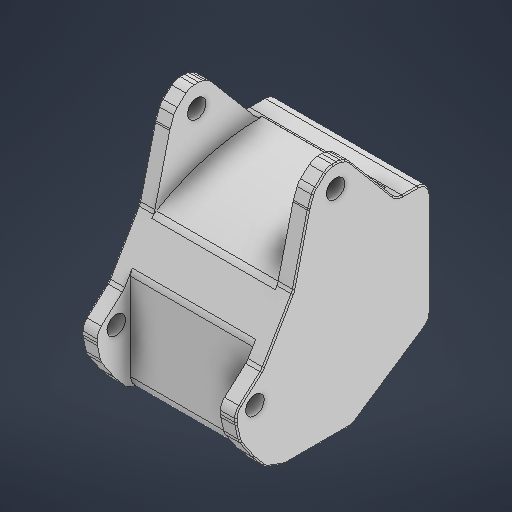
# Autodesk Inventor part: bas
Saved by Autodesk Inventor 2026 (Build 300175000, 175)
## iProperties
Created: 2025-04-29
Part Number: bas
Material: Generic
Document SubType Name: Modeling
Designer: elias
Density: 1 g/cm^3
Appearance: Default
Author: elias
Autodesk Inventor part; units mm, degrees
ref_plane "YZ Plane" through (0, 0, 0) normal (1, 0, 0) x (0, 1, 0)
ref_plane "XZ Plane" through (0, 0, 0) normal (0, 1, 0) x (-1, 0, 0)
ref_plane "XY Plane" through (0, 0, 0) normal (0, 0, 1) x (1, 0, 0)
sketch "Sketch1" plane through (0, 0, 0) normal (1, 0, 0) x (0, 1, 0)
  line L0 (3056.2025, 0) -> (3056.2025, -6694.5386) construction
  line L1 (3056.2025, -6694.5386) -> (0, -6694.5386) construction
  line L2 (0, -6694.5386) -> (0, 0) construction
  line L3 (0, 0) -> (3056.2025, 0) construction
  point P0 (0, 0)
  constraints: 2 end point, 2 other
sketch "Sketch3" plane through (0, 0, 0) normal (1, 0, 0) x (0, 1, 0)
  line L0 (685.9944, -4625.4625) -> (724.6137, -4668.6643)
  line L1 (724.6137, -4668.6643) -> (809.1123, -4718.3258)
  line L2 (809.1123, -4718.3258) -> (912.0878, -4743.403)
  line L3 (912.0878, -4743.403) -> (934.1067, -4751.4736)
  line L4 (934.1067, -4751.4736) -> (945.5061, -4764.2256)
  line L5 (945.5061, -4764.2256) -> (955.4629, -4775.3639)
  line L6 (955.4629, -4775.3639) -> (955.4629, -4793.4979)
  line L7 (955.4629, -4793.4979) -> (950.4845, -4807.0804)
  line L8 (950.4845, -4807.0804) -> (855.8729, -4886.5328)
  line L9 (855.8729, -4886.5328) -> (855.8729, -4940.715)
  line L10 (855.8729, -4940.715) -> (817.0202, -4940.715)
  line L11 (817.0202, -4940.715) -> (659.1622, -4940.715)
  line L12 (659.1622, -4940.715) -> (574.4497, -4814.0948)
  line L13 (574.4497, -4814.0948) -> (574.4497, -4703.7938)
  line L14 (574.4497, -4703.7938) -> (585.6108, -4673.3431)
  line L15 (585.6108, -4673.3431) -> (609.1892, -4653.5426)
  line L16 (609.1892, -4653.5426) -> (641.8589, -4631.6856)
  line L17 (641.8589, -4631.6856) -> (669.5109, -4625.4625)
  line L18 (669.5109, -4625.4625) -> (685.9944, -4625.4625)
  circle A0 centre (681.295, -4656.3748) radius 15
  circle A1 centre (920.0279, -4787.0013) radius 15
  point P0 (0, 0)
  dimension "d14" = 30
  dimension "d15" = 30
  constraints: 38 end point, 5 perpendicular, 4 parallel, 2 centre point, 2 point on line, 1 vertical
  measures "d14" diameter of A0
  measures "d15" diameter of A1
extrude "Extrusion1" add sketch "Sketch3" along normal mid plane 250
fillet "Fillet1" radius 20 17 edges at (0, 669.5109, -4625.4625) (0, 685.9944, -4625.4625) (0, 724.6137, -4668.6643) (0, 809.1123, -4718.3258) (0, 912.0878, -4743.403) (0, 934.1067, -4751.4736) (0, 950.4845, -4807.0804) (0, 955.4629, -4793.4979) (0, 955.4629, -4775.3639) (0, 855.8729, -4886.5328) (0, 855.8729, -4940.715) (0, 659.1622, -4940.715) (0, 574.4497, -4814.0948) (0, 641.8589, -4631.6856) (0, 609.1892, -4653.5426) (0, 585.6108, -4673.3431) (0, 574.4497, -4703.7938)
fillet "Fillet2" radius 2 68 edges at (125, 724.7675, -4668.4766) (125, 707.2443, -4649.2338) (125, 685.2143, -4627.2062) (125, 674.3902, -4625.4625) (125, 669.5245, -4625.5849) (125, 656.4177, -4628.4091) (125, 641.9946, -4632.0016) (125, 624.4291, -4643.3467) (125, 609.207, -4653.5663) (125, 599.0237, -4662.0793) (125, 586.1824, -4673.7441) (125, 579.7239, -4689.4044) (125, 574.7575, -4703.8485) (125, 574.4497, -4757.6826) (125, 575.3126, -4813.8328) (125, 615.5244, -4875.4894) (125, 660.4221, -4938.3562) (125, 752.8589, -4940.715) (125, 850.015, -4934.8572) (125, 855.8729, -4908.2846) (125, 857.745, -4887.4053) (125, 904.7067, -4845.5234) (125, 949.913, -4806.6794) (125, 953.2801, -4799.4532) (125, 955.1551, -4793.4433) (125, 955.4629, -4786.474) (125, 954.1474, -4775.8662) (125, 943.9066, -4762.4363) (125, 933.761, -4751.983) (125, 921.2781, -4746.7715) (125, 912.0786, -4743.4333) (125, 861.4842, -4731.0797) (125, 809.1934, -4718.1258) (125, 766.9404, -4693.5405) (-125, 912.0786, -4743.4333) (-125, 921.2781, -4746.7715) (-125, 933.761, -4751.983) (-125, 943.9066, -4762.4363) (-125, 954.1474, -4775.8662) (-125, 955.4629, -4786.474) (-125, 955.1551, -4793.4433) (-125, 953.2801, -4799.4532) (-125, 949.913, -4806.6794) (-125, 904.7067, -4845.5234) (-125, 857.745, -4887.4053) (-125, 855.8729, -4908.2846) (-125, 850.015, -4934.8572) (-125, 752.8589, -4940.715) (-125, 660.4221, -4938.3562) (-125, 615.5244, -4875.4894) (-125, 575.3126, -4813.8328) (-125, 574.4497, -4757.6826) (-125, 574.7575, -4703.8485) (-125, 579.7239, -4689.4044) (-125, 586.1824, -4673.7441) (-125, 599.0237, -4662.0793) (-125, 609.207, -4653.5663) (-125, 624.4291, -4643.3467) (-125, 641.9946, -4632.0016) (-125, 656.4177, -4628.4091) (-125, 669.5245, -4625.5849) (-125, 674.3902, -4625.4625) (-125, 685.2143, -4627.2062) (-125, 707.2443, -4649.2338) (-125, 724.7675, -4668.4766) (-125, 766.9404, -4693.5405) (-125, 809.1934, -4718.1258) (-125, 861.4842, -4731.0797)
sketch "Sketch4" plane through (0, 0, 0) normal (1, 0, 0) x (0, 1, 0)
  line L0 (855.8729, -4920.715) -> (855.8729, -4895.8541) projected
  arc A0 (806.5728, -4716.8332) -> (811.9744, -4719.0227) centre (816.7066, -4699.5907) ccw projected
  arc A1 (855.8729, -4895.8541) -> (806.5728, -4716.8332) centre (511.0401, -4894.5179) ccw
  line L1 (967.3012, -4716.8332) -> (967.3012, -4894.5179)
  line L2 (967.3012, -4894.5179) -> (855.8729, -4893.1817)
  line L3 (806.5728, -4716.8332) -> (727.308, -4670.2478) projected
  line L4 (743.5882, -4679.816) -> (565.7197, -4679.816)
  line L5 (565.7197, -4679.816) -> (565.7197, -4582.24)
  line L6 (565.7197, -4582.24) -> (806.5728, -4582.24)
  line L7 (806.5728, -4582.24) -> (967.3012, -4716.8332)
  line L8 (743.5882, -4679.816) -> (775.0066, -4679.816)
  line L9 (775.0066, -4679.816) -> (806.5728, -4716.8332)
  point P0 (0, 0)
  constraints: 16 end point, 3 point on circle, 3 point on line, 2 perpendicular, 1 centre point, 1 horizontal
extrude "Extrusion2" cut sketch "Sketch4" along normal mid plane 200 contours A1 L9 L8 L4 L5 L6 L7 L1 L2
fillet "Fillet3" radius 20 2 edges at (0, 806.5728, -4716.8332) (0, 743.5882, -4679.816)
fillet "Fillet4" radius 20 1 edges at (0, 583.2383, -4679.816)
body "Solid1"
